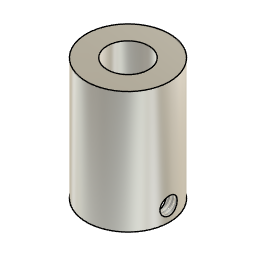
MRG25-8-12 (Autodesk Fusion 360 design; units mm, degrees)
Autodesk Fusion 360 part; units mm, degrees
sketch "スケッチ1" plane through (0, 0, 0) normal (0, 0, 1) x (1, 0, 0)
  circle A0 centre (0, 0) radius 12.5
  dimension "d1" = 25
  constraint coincident A0.centre origin
  measures "d1" diameter of A0
extrude "押し出し1" add sketch "スケッチ1" along normal blind 36
sketch "スケッチ2" plane through (0, 0, 36) normal (0, 0, 1) x (-1, 0, 0)
  circle A0 centre (0, 0) radius 12.5
  circle A1 centre (0, 0) radius 4
  dimension "d4" = 8
  constraint coincident A0.centre A1.centre
  measures "d4" diameter of A1
extrude "押し出し2" cut sketch "スケッチ2" against normal blind 18 contours A1
sketch "スケッチ3" plane through (0, 0, 0) normal (0, 0, -1) x (1, 0, 0)
  circle A0 centre (0, 0) radius 12.5
  circle A1 centre (0, 0) radius 6
  dimension "d7" = 12
  constraint concentric A0 A1
  measures "d7" diameter of A1
extrude "押し出し3" cut sketch "スケッチ3" against normal blind 18 contours A1
sketch "スケッチ4" plane through (0, 0, 36) normal (0, 0, 1) x (-1, 0, 0)
  circle A0 centre (0, 0) radius 4
  circle A1 centre (0, 0) radius 12.5
  circle A2 centre (0, 0) radius 8
  dimension "d10" = 16
  constraint coincident A0.centre A1.centre
  measures "d10" diameter of A2
extrude "押し出し4" cut sketch "スケッチ4" against normal blind 36 contours A1
extrude "押し出し5" cut 1 faces at (-7.2812, 0.6955, 0) along direction (0, 0, 1) blind 12.5
move_body "移動1" bodies 1 to x (1, 0, 0) y (0, 1, 0) z (0, 0, 1) at (0, 0, -12.5)
sketch "スケッチ5" plane through (0, 0, 0) normal (1, 0, 0) x (0, 1, 0)
  line L0 (0, 0) -> (0, 2.75)
  circle A0 centre (0, 2.75) radius 2
  dimension "d15" = 2.75
  dimension "d16" = 4
  constraint coincident L0.start origin
  constraint vertical L0
  constraint coincident L0.end A0.centre
  measures "d15" distance of L0.start L0.end
  measures "d16" diameter of A0
extrude "押し出し6" cut sketch "スケッチ5" along normal blind 8.5
thread "ねじ1" "ISO Metric profile 4.0 M4x0.7 6H" major diameter 4.1095 minor diameter 3.332 pitch 0.7 angle 60 resizes the face on face at (6.6211, -0.7665, 0.9027)
sketch "スケッチ6" plane through (0, 0, 0) normal (0, 1, 0) x (1, 0, 0)
  line L0 (0, 0) -> (0, -2.75)
  circle A0 centre (0, -2.75) radius 2
  dimension "d21" = 2.75
  dimension "d22" = 4
  constraint coincident L0.start origin
  constraint vertical L0
  constraint coincident L0.end A0.centre
  measures "d21" distance of L0.start L0.end
  measures "d22" diameter of A0
extrude "押し出し7" cut sketch "スケッチ6" along normal blind 8
thread "ねじ2" "ISO Metric profile 4.0 M4x0.7 6H" major diameter 4.1095 minor diameter 3.332 pitch 0.7 angle 60 resizes the face on face at (0.693, 7.2999, 0.8739)
